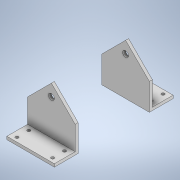
# Autodesk Inventor part: Intake - Piston Mounting Brackets
Saved by Autodesk Inventor 2020 (Build 240168000, 168)
## iProperties
Created: 2020-02-05
Part Number: Intake - Piston Mounting Brackets
Material: Generic
Document SubType Name: Modeling
Designer: aidan
Density: 1 g/cm^3
Appearance: Default
Author: aidan
Autodesk Inventor part; units mm, degrees
ref_plane "YZ Plane" through (0, 0, 0) normal (1, 0, 0) x (0, 1, 0)
ref_plane "XZ Plane" through (0, 0, 0) normal (0, 1, 0) x (-1, 0, 0)
sketch "Sketch1" plane through (0, 0, 0) normal (0, 1, 0) x (-1, 0, 0)
  line L0 (0, 0) -> (50.8, 0)
  line L1 (50.8, 0) -> (50.8, -25.4)
  line L2 (50.8, -25.4) -> (0, -25.4)
  line L3 (0, -25.4) -> (0, 0)
  dimension "d0" = 50.8
  dimension "d1" = 25.4
  constraints: 8 end point, 2 parallel, 1 horizontal, 1 perpendicular
  measures "d0" distance of L1.end L2.end
  measures "d1" distance of L0.end L1.end
extrude "Extrusion1" add sketch "Sketch1" along normal blind 3.175
sketch "Sketch2" plane through (0, 3.175, 0) normal (0, 1, 0) x (1, 0, 0)
  line L0 (0, 0) -> (0, 25.4) projected
  line L1 (-50.8, 25.4) -> (-50.8, 0) projected
  line L2 (0, 25.4) -> (-50.8, 25.4)
  line L3 (-50.8, 25.4) -> (-50.8, 22.225)
  line L4 (-50.8, 22.225) -> (0, 22.225)
  line L5 (0, 22.225) -> (0, 25.4)
  dimension "d4" = 3.175
  constraints: 8 end point, 2 parallel, 1 horizontal, 1 perpendicular, 1 point on line
  measures "d4" distance of L3.end L2.end
extrude "Extrusion2" add sketch "Sketch2" along normal blind 25.4
sketch "Sketch3" plane through (-50.8, 3.175, -22.225) normal (0, 0, 1) x (1, 0, 0)
  line L0 (0, -3.175) -> (0, 25.4) projected
  line L1 (50.8, 25.4) -> (0, 25.4) projected
  line L2 (0, 25.4) -> (50.8, 25.4)
  line L3 (50.8, 25.4) -> (25.4, 50.8)
  line L4 (25.4, 50.8) -> (0, 25.4)
  point P0 (50.8, -3.175)
  dimension "d7" = 25.4
  constraints: 6 end point, 1 collinear, 1 perpendicular
  measures "d7" distance from line of L1 L3.end
extrude "Extrusion3" add sketch "Sketch3" against normal blind 3.175
sketch "Sketch4" plane through (-50.8, 3.175, -22.225) normal (0, 0, 1) x (1, 0, 0)
  circle A0 centre (25.4, 38.1) radius 3.175
  point P0 (50.8, -3.175)
  point P1 (25.4, 50.8)
  dimension "d10" = 6.35
  dimension "d11" = 12.7
  constraints: 1 centre point, 1 vertical alignment
  measures "d10" diameter of A0
  measures "d11" distance of point (25.4, 50.8) A0.centre
extrude "Extrusion4" cut sketch "Sketch4" against normal blind 3.175
sketch "Sketch5" plane through (0, 3.175, 0) normal (0, 1, 0) x (1, 0, 0)
  line L0 (-44.45, 4.445) -> (-6.35, 4.445)
  line L1 (-6.35, 4.445) -> (-6.35, 17.145)
  line L2 (-6.35, 17.145) -> (-44.45, 17.145)
  line L3 (-44.45, 17.145) -> (-44.45, 4.445)
  line L4 (-50.8, 0) -> (0, 0) projected
  line L5 (-50.8, 22.225) -> (-50.8, 0) projected
  dimension "d14" = 38.1
  dimension "d15" = 12.7
  dimension "d16" = 4.445
  dimension "d17" = 6.35
  constraints: 8 end point, 2 parallel, 1 horizontal, 1 perpendicular
  measures "d14" distance of L2.end L1.end
  measures "d15" distance of L1.end L0.end
  measures "d16" distance between parallel lines of L4 L0
  measures "d17" distance between parallel lines of L5 L3
hole "Hole1" at (-44.45, 3.175, -17.145) at (-6.35, 3.175, -17.145) at (-6.35, 3.175, -4.445) at (-44.45, 3.175, -4.445) direction (0, -1, 0) diameter 3.175 end through all
ref_plane "Work Plane1" through (0, 0, -63.5) normal (0, 0, -1) x (-1, 0, 0)
mirror "Mirror1" about plane through (0, 0, -63.5) normal (0, 0, -1)
body "Solid1"
